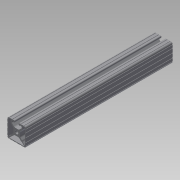
# Autodesk Inventor part: 1501
Saved by Autodesk Inventor 2013 (Build 170138000, 138)
## iProperties
Created: 2014-04-23
Part Number: 1501
Material: Generic
Document SubType Name: Modeling
Density: 1 g/cm^3
Vendor: 80/20 Inc.
Engineer: Ross Bowman
Designer: Ross Bowman
Catalog Web Link: 8020.net
Company: 80/20 Inc.
Author: Ross Bowman
Keywords: 80/20 , 8020 , T-Slot , Extrusion
Material: 6105-T5 Aluminum
Autodesk Inventor part; units mm, degrees
ref_plane "YZ Plane" through (0, 0, 0) normal (1, 0, 0) x (0, 1, 0)
ref_plane "XZ Plane" through (0, 0, 0) normal (0, 1, 0) x (-1, 0, 0)
ref_plane "XY Plane" through (0, 0, 0) normal (0, 0, 1) x (1, 0, 0)
sketch "Sketch1" plane through (0, 0, 0) normal (0, 0, 1) x (1, 0, 0)
  arc A0 (11.091, -12.3537) -> (10.924, -12.2274) centre (10.5522, -12.8925) ccw
  line L0 (15.3589, -16.6216) -> (11.091, -12.3537)
  arc A1 (15.0895, -17.272) -> (15.3589, -16.6216) centre (15.0895, -16.891) ccw
  line L1 (-15.0895, -17.272) -> (15.0895, -17.272)
  arc A2 (-15.3589, -16.6216) -> (-15.0895, -17.272) centre (-15.0895, -16.891) ccw
  line L2 (-11.091, -12.3537) -> (-15.3589, -16.6216)
  arc A3 (-10.924, -12.2274) -> (-11.091, -12.3537) centre (-10.5522, -12.8925) ccw
  line L3 (-9.0722, -11.1921) -> (-10.924, -12.2274)
  arc A4 (-9.0722, -11.1921) -> (-8.9052, -11.0658) centre (-9.4441, -10.527) ccw
  line L4 (-6.1016, -8.262) -> (-8.9052, -11.0658)
  arc A5 (-2.7429, -6.8707) -> (-6.1016, -8.262) centre (-2.7429, -11.6205) ccw
  line L5 (2.7429, -6.8707) -> (-2.7429, -6.8707)
  arc A6 (6.1016, -8.262) -> (2.7429, -6.8707) centre (2.7429, -11.6205) ccw
  line L6 (8.9052, -11.0658) -> (6.1016, -8.262)
  arc A7 (8.9052, -11.0658) -> (9.0722, -11.1921) centre (9.4441, -10.527) ccw
  line L7 (10.924, -12.2274) -> (9.0722, -11.1921)
  arc A8 (-12.1736, 16.891) -> (-12.5546, 17.272) centre (-12.5546, 16.891) ccw
  line L8 (-12.1736, 11.2243) -> (-12.1736, 16.891)
  arc A9 (-12.1736, 11.2243) -> (-11.2435, 8.979) centre (-8.9986, 11.2243) ccw
  line L9 (-8.1479, 5.8839) -> (-11.2435, 8.979)
  arc A10 (-6.7564, 2.525) -> (-8.1479, 5.8839) centre (-11.5062, 2.525) ccw
  line L10 (-6.7564, -2.6388) -> (-6.7564, 2.525)
  arc A11 (-8.1475, -5.9974) -> (-6.7564, -2.6388) centre (-11.5062, -2.6388) ccw
  line L11 (-10.9781, -8.8281) -> (-8.1475, -5.9974)
  arc A12 (-10.9781, -8.8281) -> (-11.1044, -8.9951) centre (-10.4393, -9.3669) ccw
  line L12 (-12.14, -10.8475) -> (-11.1044, -8.9951)
  arc A13 (-12.2663, -11.0145) -> (-12.14, -10.8475) centre (-12.8051, -10.4757) ccw
  line L13 (-16.6875, -15.4357) -> (-12.2663, -11.0145)
  arc A14 (-17.272, -15.1936) -> (-16.6875, -15.4357) centre (-16.9296, -15.1936) ccw
  line L14 (-17.272, 14.478) -> (-17.272, -15.1936)
  arc A15 (-14.478, 17.272) -> (-17.272, 14.478) centre (-14.478, 14.478) ccw
  line L15 (-12.5546, 17.272) -> (-14.478, 17.272)
  arc A16 (17.272, 14.478) -> (14.478, 17.272) centre (14.478, 14.478) ccw
  line L16 (17.272, -15.1936) -> (17.272, 14.478)
  arc A17 (16.6875, -15.4357) -> (17.272, -15.1936) centre (16.9296, -15.1936) ccw
  line L17 (12.2663, -11.0145) -> (16.6875, -15.4357)
  arc A18 (12.14, -10.8475) -> (12.2663, -11.0145) centre (12.8051, -10.4757) ccw
  line L18 (11.1044, -8.9951) -> (12.14, -10.8475)
  arc A19 (11.1044, -8.9951) -> (10.9781, -8.8281) centre (10.4393, -9.3669) ccw
  line L19 (8.1475, -5.9974) -> (10.9781, -8.8281)
  arc A20 (6.7564, -2.6388) -> (8.1475, -5.9974) centre (11.5062, -2.6388) ccw
  line L20 (6.7564, 2.525) -> (6.7564, -2.6388)
  arc A21 (8.1479, 5.8839) -> (6.7564, 2.525) centre (11.5062, 2.525) ccw
  line L21 (11.2435, 8.979) -> (8.1479, 5.8839)
  arc A22 (11.2435, 8.979) -> (12.1736, 11.2243) centre (8.9986, 11.2243) ccw
  line L22 (12.1736, 16.891) -> (12.1736, 11.2243)
  arc A23 (12.5546, 17.272) -> (12.1736, 16.891) centre (12.5546, 16.891) ccw
  line L23 (14.478, 17.272) -> (12.5546, 17.272)
  circle A24 centre (0, 0) radius 3.3274
  line L24 (6.8141, 14.986) -> (6.8141, 15.8247)
  line L25 (6.8141, 15.8247) -> (9.017, 15.8247)
  arc A25 (10.287, 14.5547) -> (9.017, 15.8247) centre (9.017, 14.5547) ccw
  line L26 (10.287, 14.5547) -> (10.287, 12.8154)
  arc A26 (10.0266, 12.1868) -> (10.287, 12.8154) centre (9.398, 12.8154) ccw
  line L27 (10.0266, 12.1868) -> (6.1008, 8.2616)
  arc A27 (2.7424, 6.8707) -> (6.1008, 8.2616) centre (2.7424, 11.6205) ccw
  line L28 (2.7424, 6.8707) -> (-2.7424, 6.8707)
  arc A28 (-6.1008, 8.2616) -> (-2.7424, 6.8707) centre (-2.7424, 11.6205) ccw
  line L29 (-6.1008, 8.2616) -> (-10.0266, 12.1868)
  arc A29 (-10.287, 12.8154) -> (-10.0266, 12.1868) centre (-9.398, 12.8154) ccw
  line L30 (-10.287, 12.8154) -> (-10.287, 14.5547)
  arc A30 (-9.017, 15.8247) -> (-10.287, 14.5547) centre (-9.017, 14.5547) ccw
  line L31 (-9.017, 15.8247) -> (-6.8141, 15.8247)
  line L32 (-6.8141, 15.8247) -> (-6.8141, 14.986)
  line L33 (-6.8141, 14.986) -> (-5.6388, 14.986)
  arc A31 (-5.6388, 14.986) -> (-4.064, 16.5608) centre (-5.6388, 16.5608) ccw
  line L34 (-4.064, 16.5608) -> (-4.064, 17.4752)
  arc A32 (-4.064, 17.4752) -> (-5.6388, 19.05) centre (-5.6388, 17.4752) ccw
  line L35 (-5.6388, 19.05) -> (-7.9756, 19.05)
  arc A33 (-9.4996, 19.05) -> (-7.9756, 19.05) centre (-8.7376, 19.05) ccw
  line L36 (-9.4996, 19.05) -> (-14.3256, 19.05)
  arc A34 (-15.8496, 19.05) -> (-14.3256, 19.05) centre (-15.0876, 19.05) ccw
  line L37 (-15.8496, 19.05) -> (-15.875, 19.05)
  arc A35 (-15.875, 19.05) -> (-19.05, 15.875) centre (-15.875, 15.875) ccw
  line L38 (-19.05, 15.875) -> (-19.05, 15.8496)
  arc A36 (-19.05, 14.3256) -> (-19.05, 15.8496) centre (-19.05, 15.0876) ccw
  line L39 (-19.05, 14.3256) -> (-19.05, 9.4996)
  arc A37 (-19.05, 7.9756) -> (-19.05, 9.4996) centre (-19.05, 8.7376) ccw
  line L40 (-19.05, 7.9756) -> (-19.05, 0.762)
  arc A38 (-19.05, -0.762) -> (-19.05, 0.762) centre (-19.05, 0) ccw
  line L41 (-19.05, -0.762) -> (-19.05, -7.9756)
  arc A39 (-19.05, -9.4996) -> (-19.05, -7.9756) centre (-19.05, -8.7376) ccw
  line L42 (-19.05, -9.4996) -> (-19.05, -14.3256)
  arc A40 (-19.05, -15.8496) -> (-19.05, -14.3256) centre (-19.05, -15.0876) ccw
  line L43 (-19.05, -15.8496) -> (-19.05, -15.875)
  arc A41 (-19.05, -15.875) -> (-15.875, -19.05) centre (-15.875, -15.875) ccw
  line L44 (-15.875, -19.05) -> (-15.8496, -19.05)
  arc A42 (-14.3256, -19.05) -> (-15.8496, -19.05) centre (-15.0876, -19.05) ccw
  line L45 (-14.3256, -19.05) -> (-9.4996, -19.05)
  arc A43 (-7.9756, -19.05) -> (-9.4996, -19.05) centre (-8.7376, -19.05) ccw
  line L46 (-7.9756, -19.05) -> (-0.762, -19.05)
  arc A44 (0.762, -19.05) -> (-0.762, -19.05) centre (0, -19.05) ccw
  line L47 (0.762, -19.05) -> (7.9756, -19.05)
  arc A45 (9.4996, -19.05) -> (7.9756, -19.05) centre (8.7376, -19.05) ccw
  line L48 (9.4996, -19.05) -> (14.3256, -19.05)
  arc A46 (15.8496, -19.05) -> (14.3256, -19.05) centre (15.0876, -19.05) ccw
  line L49 (15.8496, -19.05) -> (15.875, -19.05)
  arc A47 (15.875, -19.05) -> (19.05, -15.875) centre (15.875, -15.875) ccw
  line L50 (19.05, -15.875) -> (19.05, -15.8496)
  arc A48 (19.05, -14.3256) -> (19.05, -15.8496) centre (19.05, -15.0876) ccw
  line L51 (19.05, -14.3256) -> (19.05, -9.4996)
  arc A49 (19.05, -7.9756) -> (19.05, -9.4996) centre (19.05, -8.7376) ccw
  line L52 (19.05, -7.9756) -> (19.05, -0.762)
  arc A50 (19.05, 0.762) -> (19.05, -0.762) centre (19.05, 0) ccw
  line L53 (19.05, 0.762) -> (19.05, 7.9756)
  arc A51 (19.05, 9.4996) -> (19.05, 7.9756) centre (19.05, 8.7376) ccw
  line L54 (19.05, 9.4996) -> (19.05, 14.3256)
  arc A52 (19.05, 15.8496) -> (19.05, 14.3256) centre (19.05, 15.0876) ccw
  line L55 (19.05, 15.8496) -> (19.05, 15.875)
  arc A53 (19.05, 15.875) -> (15.875, 19.05) centre (15.875, 15.875) ccw
  line L56 (15.875, 19.05) -> (15.8496, 19.05)
  arc A54 (14.3256, 19.05) -> (15.8496, 19.05) centre (15.0876, 19.05) ccw
  line L57 (14.3256, 19.05) -> (9.4996, 19.05)
  arc A55 (7.9756, 19.05) -> (9.4996, 19.05) centre (8.7376, 19.05) ccw
  line L58 (7.9756, 19.05) -> (5.6388, 19.05)
  arc A56 (5.6388, 19.05) -> (4.064, 17.4752) centre (5.6388, 17.4752) ccw
  line L59 (4.064, 17.4752) -> (4.064, 16.5608)
  arc A57 (4.064, 16.5608) -> (5.6388, 14.986) centre (5.6388, 16.5608) ccw
  line L60 (5.6388, 14.986) -> (6.8141, 14.986)
  constraints: 122 end point, 114 point on circle, 58 centre point
extrude "Extrusion1" add sketch "Sketch1" against normal blind 304.8
body "Solid1"
